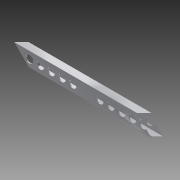
# Autodesk Inventor part: rail support 2x1
Saved by Autodesk Inventor 2015 SP1 (Build 190203100, 203)
## iProperties
Created: 2015-01-26
Part Number: rail support 2x1
Material: Aluminum 6061
Document SubType Name: Modeling
Designer: Admin
Density: 2.7 g/cm^3
Appearance: Aluminum - Flat
Author: Admin
Autodesk Inventor part; units mm, degrees
ref_plane "YZ Plane" through (0, 0, 0) normal (1, 0, 0) x (0, 1, 0)
ref_plane "XZ Plane" through (0, 0, 0) normal (0, 1, 0) x (-1, 0, 0)
ref_plane "XY Plane" through (0, 0, 0) normal (0, 0, 1) x (1, 0, 0)
sketch "Sketch1" plane through (0, 0, 0) normal (1, 0, 0) x (0, 1, 0)
  line L0 (0, 0) -> (-50.8, 0)
  line L1 (-50.8, 0) -> (-50.8, -25.4)
  line L2 (-50.8, -25.4) -> (0, -25.4)
  line L3 (0, -25.4) -> (0, 0)
  line L4 (-3.175, -3.175) -> (-47.625, -3.175)
  line L5 (-47.625, -3.175) -> (-47.625, -22.225)
  line L6 (-47.625, -22.225) -> (-3.175, -22.225)
  line L7 (-3.175, -22.225) -> (-3.175, -3.175)
  dimension "d0" = 50.8
  dimension "d1" = 25.4
  dimension "d2" = 44.45
  dimension "d3" = 19.05
  dimension "d4" = 3.175
  dimension "d5" = 3.175
  constraints: 16 end point, 4 parallel, 2 horizontal, 2 perpendicular
  measures "d0" distance of L2.end L1.end
  measures "d1" distance of L1.end L0.end
  measures "d2" distance of L6.end L5.end
  measures "d3" distance between parallel lines of L6 L4
  measures "d4" distance between parallel lines of L0 L4
  measures "d5" distance between parallel lines of L3 L7
extrude "Extrusion1" add sketch "Sketch1" along normal blind 552.45
fillet "Fillet1" radius 3.175 2 edges at (0, -50.8, -12.7) (552.45, -50.8, -12.7)
sketch "Sketch4" plane through (0, 0, 0) normal (0, 0, 1) x (1, 0, 0)
  line L0 (0, 0) -> (552.45, 0) projected
  line L1 (0, 0) -> (0, -47.625) projected
  point P0 (76.2, -25.4)
  dimension "d33" = 25.4
  dimension "d34" = 76.2
  measures "d33" distance from line of L0 point (76.2, -25.4)
  measures "d34" distance from line of L1 point (76.2, -25.4)
hole "Hole3" at (76.2, -25.4, 0) direction (0, 0, -1) diameter 25.4 end through all
pattern_linear "Rectangular Pattern3" count 5 spacing 38.1 along (1, 0, 0) of "Hole3"
sketch "Sketch5" plane through (0, 0, 0) normal (0, 0, 1) x (1, 0, 0)
  line L0 (552.45, 0) -> (552.45, -47.625) projected
  line L1 (0, 0) -> (552.45, 0) projected
  point P0 (476.25, -25.4)
  dimension "d45" = 76.2
  dimension "d46" = 25.4
  measures "d45" distance from line of L0 point (476.25, -25.4)
  measures "d46" distance from line of L1 point (476.25, -25.4)
hole "Hole4" at (476.25, -25.4, 0) direction (0, 0, -1) diameter 25.4 end through all
pattern_linear "Rectangular Pattern4" count 5 spacing 38.1 along (-1, 0, 0) of "Hole4"
body "Solid1"
